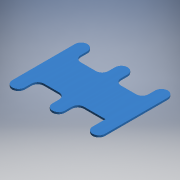
# Autodesk Inventor part: Body_bottom
Saved by Autodesk Inventor 2017 (Build 210142000, 142)
## iProperties
Part Number: Body_bottom
Material: Generic
Document SubType Name: Modeling
Designer: alex-
Appearance: Cyan
Author: alex-
Autodesk Inventor part; units mm, degrees
ref_plane "YZ Plane" through (0, 0, 0) normal (1, 0, 0) x (0, 1, 0)
ref_plane "XZ Plane" through (0, 0, 0) normal (0, 1, 0) x (-1, 0, 0)
ref_plane "XY Plane" through (0, 0, 0) normal (0, 0, 1) x (1, 0, 0)
sketch "Sketch1" plane through (0, 0, 0) normal (0, 1, 0) x (-1, 0, 0)
  line L0 (126, 102) -> (92, 102)
  line L1 (126, -102) -> (92, -102)
  line L2 (126, 102) -> (126, -102)
  line L3 (92, 102) -> (92, 50)
  line L4 (92, -50) -> (92, -102)
  line L5 (92, 50) -> (17, 50)
  line L6 (92, -50) -> (17, -50)
  line L7 (17, 50) -> (17, 102)
  line L8 (17, -50) -> (17, -102)
  line L9 (17, 102) -> (-17, 102)
  line L10 (17, -102) -> (-17, -102)
  line L11 (-17, 102) -> (-17, 50)
  line L12 (-17, -50) -> (-17, -102)
  line L13 (-17, 50) -> (-92, 50)
  line L14 (-17, -50) -> (-92, -50)
  line L15 (-92, 50) -> (-92, 102)
  line L16 (-92, -50) -> (-92, -102)
  line L17 (-92, 102) -> (-126, 102)
  line L18 (-92, -102) -> (-126, -102)
  line L19 (-126, 102) -> (-126, -102)
  line L20 (126, 0) -> (-126, 0) construction
  line L21 (0, 102) -> (0, -102) construction
  point P0 (0, 0)
  point P1 (0, 0)
  dimension "d0" = 204
  dimension "d1" = 34
  dimension "d3" = 75
  dimension "d4" = 52
  dimension "d5" = 100
  constraints: 44 end point, 16 equal length, 9 vertical, 8 horizontal, 6 horizontal alignment, 5 midpoint, 1 coincident, 1 parallel, 1 perpendicular
  measures "d0" distance of L0.start L1.start
  measures "d1" distance of L0.start L0.end
  measures "d3" distance of L3.end L5.end
  measures "d4" distance of L0.end L3.end
  measures "d5" distance between parallel lines of L6 L5
extrude "Extrusion1" add sketch "Sketch1" along normal blind 5
fillet "Fillet1" radius 17 19 edges at (-126, 2.5, 102) (-92, 2.5, 102) (-92, 2.5, 50) (92, 2.5, 102) (126, 2.5, 102) (17, 2.5, 102) (-17, 2.5, 102) (17, 2.5, 50) (-17, 2.5, 50) (-126, 2.5, -102) (-92, 2.5, -102) (-17, 2.5, -50) (-17, 2.5, -102) (17, 2.5, -102) (92, 2.5, -50) (92, 2.5, -102) (126, 2.5, -102) (17, 2.5, -50) (-92, 2.5, -50)
equation "\"d1\" = sa_diameter + 2 * b_mat_thickness"
equation "\"d3\" = b_leg_space"
equation "\"d4\" = s_land + s_width + b_mat_thickness"
equation "\"d5\" = b_core_width"
equation "\"d6\" = b_mat_thickness"
equation "\"d22\" = b_mat_thickness + 0.5 * sa_diameter"
equation "\"sa_diameter\" = 24"
equation "\"b_mat_thickness\" = 5"
equation "\"b_leg_space\" = 75"
equation "\"s_land\" = 6.5"
equation "\"s_width\" = 40.5"
equation "\"b_core_width\" = 100"
body "Solid1"
